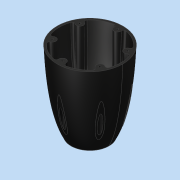
# Autodesk Inventor part: foreHullLower
Saved by Autodesk Inventor 2017 (Build 210142000, 142)
## iProperties
Created: 2016-09-09
Part Number: foreHullLower
Material: Generic
Document SubType Name: Modeling
Designer: techn
Density: 1 g/cm^3
Appearance: Glossy - Black
Mass: 764.223 g
Surface Area: 456.432 cm^2
Volume: 764.223 cm^3
Author: techn
Autodesk Inventor part; units mm, degrees
ref_plane "YZ Plane" through (0, 0, 0) normal (1, 0, 0) x (0, 1, 0)
ref_plane "XZ Plane" through (0, 0, 0) normal (0, 1, 0) x (-1, 0, 0)
ref_plane "XY Plane" through (0, 0, 0) normal (0, 0, 1) x (1, 0, 0)
sketch "Sketch6" plane through (0, 0, 0) normal (0, 0, 1) x (1, 0, 0)
  line L0 (540.6478, 1219.1491) -> (540.6478, -58.7076) construction
  line L1 (540.6478, -58.7076) -> (-407.4394, -58.7076) construction
  line L2 (-407.4394, -58.7076) -> (-407.4394, 1219.1491) construction
  line L3 (-407.4394, 1219.1491) -> (540.6478, 1219.1491) construction
  point P0 (0, 0)
  constraints: 2 other
sketch "Sketch5" plane through (0, 0, 0) normal (0, 0, 1) x (1, 0, 0)
  line L0 (0, 0) -> (0, 142.24)
  line L1 (0, 142.24) -> (50.8, 142.24)
  line L2 (50.8, 142.24) -> (-50.8, 142.24)
  line L3 (50.8, 142.24) -> (45.2986, 0) construction
  line L4 (45.2986, 0) -> (0, 0) construction
  spline S0 degree 2 poles (50.8, 142.24) (45.2986, 0) (0, 0) knots 1 1 1 2 2 2
  line L5 (-50.8, 142.24) -> (-45.2986, 0) construction
  line L6 (-45.2986, 0) -> (0, 0) construction
  spline S1 degree 2 poles (-50.8, 142.24) (-45.2986, 0) (0, 0) knots 1 1 1 2 2 2
  line L7 (0, 0) -> (-87.9699, 0)
  line L8 (-87.9699, 0) -> (-87.9699, 142.24)
  line L9 (-87.9699, 142.24) -> (-50.8, 142.24)
  dimension "d20" = 142.24
  dimension "d21" = 50.8
  dimension "d22" = 101.6
  constraints: 12 end point, 2 horizontal, 2 perpendicular, 1 point on line, 1 symmetric about line, 1 vertical, 6 other
  measures "d20" distance of L0.start L0.end
  measures "d21" distance of L0.end L1.end
  measures "d22" distance of L1.end L2.end
revolve "Revolution1" add sketch "Sketch5" angle 360 about axis through (0, 0, 0) along (0, 1, 0) contours L0 L1 S0
shell "Shell1" thickness 3.175 removed faces 1 at (-7.3018, 142.24, -11.5135)
ref_plane "Work Plane1" through (0, 21.59, 0) normal (0, 1, 0) x (1, 0, 0)
sketch "Sketch8" plane through (0, 21.59, 0) normal (0, 1, 0) x (1, 0, 0)
  line L0 (55.7026, -55.9089) -> (-49.7197, -55.9089)
  line L1 (-49.7197, -55.9089) -> (-49.7197, 56.7341)
  line L2 (-49.7197, 56.7341) -> (55.7026, 56.7341)
  line L3 (55.7026, 56.7341) -> (55.7026, -55.9089)
  point P0 (0, 0)
  constraints: 8 end point, 2 parallel, 1 horizontal, 1 perpendicular
extrude "Extrusion1" cut sketch "Sketch8" against normal blind 25.4
sketch "Sketch9" plane through (0, 142.24, 0) normal (0, 1, 0) x (1, 0, 0)
  line L0 (0, 0) -> (0, 42.545)
  circle A0 centre (0, 42.545) radius 1.5875
  circle A1 centre (0, 42.545) radius 3.175
  circle A2 centre (0, 42.545) radius 5.3975
  circle A3 centre (-36.8451, 21.2725) radius 5.3975
  circle A4 centre (-36.8451, 21.2725) radius 3.175
  circle A5 centre (-36.8451, 21.2725) radius 1.5875
  circle A6 centre (-36.8451, -21.2725) radius 5.3975
  circle A7 centre (-36.8451, -21.2725) radius 3.175
  circle A8 centre (-36.8451, -21.2725) radius 1.5875
  circle A9 centre (0, -42.545) radius 5.3975
  circle A10 centre (0, -42.545) radius 3.175
  circle A11 centre (0, -42.545) radius 1.5875
  circle A12 centre (36.8451, -21.2725) radius 5.3975
  circle A13 centre (36.8451, -21.2725) radius 3.175
  circle A14 centre (36.8451, -21.2725) radius 1.5875
  circle A15 centre (36.8451, 21.2725) radius 5.3975
  circle A16 centre (36.8451, 21.2725) radius 3.175
  circle A17 centre (36.8451, 21.2725) radius 1.5875
  dimension "d73" = 42.545
  dimension "d74" = 3.175
  dimension "d75" = 6.35
  dimension "d76" = 10.795
  dimension "d79" = 360
  constraints: 18 centre point, 13 coincident, 2 end point, 1 vertical, 37 other
  measures "d73" distance of L0.start L0.end
  measures "d74" diameter of A0
  measures "d75" diameter of A1
  measures "d76" diameter of A2
extrude "Extrusion2" add sketch "Sketch9" against normal blind 101.6 contours A1 | A2 | A3 | A4 | A6 | A7 | A9 | A10 | A12 | A13 | A15 | A16
ref_plane "Work Plane2" through (0, 139.065, 0) normal (0, 1, 0) x (0, 0, -1)
sketch "Sketch10" plane through (0, 139.065, 0) normal (0, 1, 0) x (0, 0, -1)
  circle A0 centre (21.2725, 36.8451) radius 1.5875 projected
  arc A1 (-47.5832, -1.9363) -> (-47.5832, 1.9363) centre (-42.545, 0) ccw projected
  arc A2 (-25.4685, 40.2402) -> (-22.1148, 42.1764) centre (-21.2725, 36.8451) ccw projected
  arc A3 (22.1148, 42.1764) -> (25.4685, 40.2402) centre (21.2725, 36.8451) ccw projected
  arc A4 (47.5832, 1.9363) -> (47.5832, -1.9363) centre (42.545, 0) ccw projected
  arc A5 (25.4685, -40.2402) -> (22.1148, -42.1764) centre (21.2725, -36.8451) ccw projected
  arc A6 (-22.1148, -42.1764) -> (-25.4685, -40.2402) centre (-21.2725, -36.8451) ccw projected
  circle A7 centre (-21.2725, 36.8451) radius 1.5875 projected
  circle A8 centre (42.545, 0) radius 1.5875 projected
  circle A9 centre (21.2725, 36.8451) radius 1.5875 projected
  circle A10 centre (-42.545, 0) radius 1.5875 projected
  circle A11 centre (21.2725, -36.8451) radius 1.5875 projected
  circle A12 centre (0, 0) radius 50.8 projected
  circle A13 centre (-21.2725, -36.8451) radius 1.5875 projected
  circle A14 centre (42.545, 0) radius 3.175
  circle A15 centre (21.2725, -36.8451) radius 3.175
  circle A16 centre (-21.2725, -36.8451) radius 3.175
  circle A17 centre (-42.545, 0) radius 3.175
  circle A18 centre (-21.2725, 36.8451) radius 3.175
  circle A19 centre (21.2725, 36.8451) radius 3.175
  point P0 (-40.7496, 24.6452)
  point P1 (-41.7182, 22.9676)
  point P2 (0, -50.8)
  dimension "d84" = 6.35
  dimension "d85" = 6.35
  dimension "d86" = 6.35
  dimension "d87" = 6.35
  dimension "d88" = 6.35
  dimension "d89" = 6.35
  constraints: 6 centre point, 6 coincident, 1 horizontal alignment, 1 vertical alignment, 7 other
  measures "d84" diameter of A14
  measures "d85" diameter of A15
  measures "d86" diameter of A16
  measures "d87" diameter of A17
  measures "d88" diameter of A18
  measures "d89" diameter of A19
extrude "Extrusion3" cut sketch "Sketch10" against normal through all contours A0 | A7 | A8 | A10 | A11 | A13 | A14 | A15 | A16 | A17 | A18 | A19
revolve "Revolution2" cut sketch "Sketch5" angle 360 about axis through (0, 0, 0) along (0, 1, 0) contours L7 L8 L9 S1
fillet "Fillet1" radius 3.175 12 edges at (-35.9312, 99.0902, -26.5921) (-40.689, 95.1856, -17.4834) (4.3482, 112.9962, -45.7429) (-5.391, 81.8904, -42.2812) (-40.6778, 95.052, 17.4721) (-35.9312, 99.09, 26.5921) (-5.393, 85.4028, 42.7646) (4.3478, 113.0017, 45.7433) (32.1495, 66.3416, 23.9342) (42.227, 138.4639, 21.6813) (42.2271, 138.4538, -21.6802) (35.2656, 59.8293, -16.1113)
body "Solid1"
